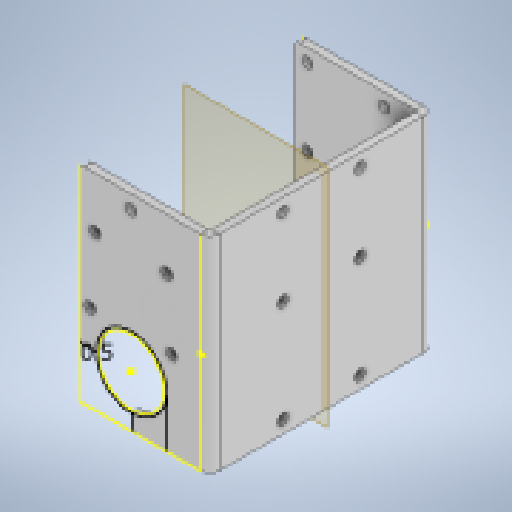
# Autodesk Inventor part: axis_3_top_frame
Saved by Autodesk Inventor 2024.1 (Build 281209000, 209)
## iProperties
Created: 2023-09-27
Part Number: axis_3_top_frame
Material: Aluminum 6061-AHC
Document SubType Name: Sheet Metal
Designer: chanh
Density: 2.7 g/cm^3
Sheet Metal Rule: Default_mm
Appearance: Aluminum - Dark
Author: chanh
Autodesk Inventor part; units mm, degrees
ref_plane "YZ Plane" through (0, 0, 0) normal (1, 0, 0) x (0, 1, 0)
ref_plane "XZ Plane" through (0, 0, 0) normal (0, 1, 0) x (-1, 0, 0)
ref_plane "XY Plane" through (0, 0, 0) normal (0, 0, 1) x (1, 0, 0)
sketch "Sketch1" plane through (0, 0, 0) normal (1, 0, 0) x (0, 1, 0)
  line L0 (20.05, 20.25) -> (-20.05, 20.25)
  line L1 (-20.05, 20.25) -> (-20.05, -20.25)
  line L2 (-20.05, -20.25) -> (20.05, -20.25)
  line L3 (20.05, -20.25) -> (20.05, 20.25)
  line L4 (20.05, 20.25) -> (-20.05, -20.25) construction
  line L5 (-20.05, 20.25) -> (20.05, -20.25) construction
  point P0 (0, 0)
  dimension "d0" = 40.1
  dimension "d1" = 40.5
  measures "d0" distance of L2.end L1.end
  measures "d1" distance of L1.end L0.end
extrude "Plate1" add sketch "Sketch1" along normal blind 1.5
sketch "Sketch2" plane through (0, 20.05, 20.25) normal (0, 0, 1) x (1, 0, 0)
  line L0 (0, -40.1) -> (0, 0)
  line L1 (0, 0) -> (-24, 0)
  line L2 (-24, 0) -> (-24, -40.1)
  line L3 (-24, -40.1) -> (0, -40.1)
  constraints: 6 end point, 1 horizontal, 1 perpendicular, 1 vertical
edge flange "Flange1" height 25.5 angle 90 thickness 1.5 bend radius 0.31 thickness toward (0, 0, 1) relief straight relief width 1.5 relief depth 0.75 corner gap 0.31 corner form 0 edges at (0, 0, 20.25) (0, 0, -20.25) wall of the first edge with corners at (0, -20.05, 20.25) (0, 20.05, 20.25) (-24, 20.05, 20.25) (-24, -20.05, 20.25)
bend "Bend1"
corner "Corner1"
sketch "Sketch3" plane through (-24, -20.05, 21.75) normal (0, 0, 1) x (1, 0, 0)
  circle A0 centre (10.07, 10) radius 6.4 projected
  line L0 (0, 0) -> (0, 40.1) projected
  line L1 (23.69, 0) -> (0, 0) projected
  line L2 (23.69, 0) -> (23.69, 40.1) projected
  circle A1 centre (10.07, 10) radius 6.9
  line L3 (3.17, 10) -> (0, 10)
  line L4 (16.97, 10) -> (16.97, 0)
  line L5 (10.07, 3.1) -> (10.07, 0)
  point P0 (24, 20.05)
  dimension "d13" = 0.5
  constraints: 6 end point, 3 point on circle, 3 point on line, 2 perpendicular, 1 centre point, 1 horizontal, 1 horizontal alignment, 1 tangent, 1 vertical alignment
  measures "d13" radial gap between concentric circles of A0 A1
sketch "Sketch4" plane through (-24, -20.05, -21.75) normal (0, 0, -1) x (-1, 0, 0)
  line L0 (-3.17, 10) -> (0, 10) projected
  line L1 (0, 0) -> (0, 40.1) projected
  circle A0 centre (-10.07, 10) radius 6.9 projected
  line L2 (-16.97, 10) -> (-16.97, 0) projected
  line L3 (-23.69, 0) -> (0, 0) projected
  line L4 (-10.07, 3.1) -> (-10.07, 0)
  point P0 (-24, 20.05)
  constraints: 2 end point, 1 perpendicular, 1 point on circle, 1 point on line, 1 vertical alignment
extrude "Cut1" cut sketch "Sketch3" against normal blind 1.5 contours A0 | L0 L3 A1 L5 L1 | A1
extrude "Cut2" cut sketch "Sketch4" against normal blind 1.5 contours A0 | L0 L1 L3 L4 A0
ref_plane "Work Plane1" through (-24, 20.05, 0) normal (0, 0, 1) x (1, 0, 0)
sketch "Sketch5" plane through (-24, 20.05, 21.75) normal (0, 0, 1) x (1, 0, 0)
  circle A0 centre (18.07, -23.2) radius 0.7835 projected
  circle A1 centre (2.07, -23.2) radius 0.7835 projected
  circle A2 centre (3.07, -9.98) radius 0.7835 projected
  circle A3 centre (17.07, -9.98) radius 0.7835 projected
  circle A4 centre (10.07, -2.68) radius 0.7835 projected
  point P0 (24, -20.05)
hole "Hole1" at (-13.93, 17.37, 21.75) at (-20.93, 10.07, 21.75) at (-6.93, 10.07, 21.75) at (-21.93, -3.15, 21.75) at (-5.93, -3.15, 21.75) direction (0, 0, -1) diameter 2.1 depth 1.5
sketch "Sketch6" plane through (-0.31, 20.05, -21.75) normal (0, 0, -1) x (-1, 0, 0)
  circle A0 centre (6.095, -17.6) radius 0.7835 projected
  circle A1 centre (6.095, -2.5) radius 0.7835 projected
  circle A2 centre (21.145, -2.5) radius 0.7835 projected
  circle A3 centre (21.145, -17.6) radius 0.7835 projected
  circle A4 centre (6.095, -37.6) radius 0.7835 projected
  point P0 (-0.31, -20.05)
fillet "Corner Round1" radius 1 6 edges at (-13.93, -20.05, -21) (-24, -10.05, -21) (-13.93, -20.05, 21) (-24, -10.05, 21) (-24, 20.05, 21) (-24, 20.05, -21)
hole "Hole3" at (-6.405, 17.55, -21.75) at (-21.455, 17.55, -21.75) at (-6.405, 2.45, -21.75) at (-21.455, 2.45, -21.75) at (-6.405, -17.55, -21.75) direction (0, 0, 1) diameter 2.1 depth 1.5
sketch "Sketch9" plane through (1.5, 0, 0) normal (1, 0, 0) x (0, 0, -1)
  circle A0 centre (7.525, 17.55) radius 0.7835
  circle A1 centre (-7.525, 17.55) radius 0.7835
  circle A2 centre (-7.525, 2.45) radius 0.7835
  circle A3 centre (7.525, 2.45) radius 0.7835
  circle A4 centre (7.525, -17.55) radius 0.7835
  circle A5 centre (-7.525, -17.55) radius 0.7835
  point P0 (0, 0)
  constraints: 6 centre point, 12 other
hole "Hole4" at (1.5, 17.55, 7.525) at (1.5, 17.55, -7.525) at (1.5, 2.45, 7.525) at (1.5, 2.45, -7.525) at (1.5, -17.55, 7.525) at (1.5, -17.55, -7.525) direction (-1, 0, 0) diameter 2.1 end through all
equation "\"d14\" = Thickness"
equation "\"d16\" = Thickness"
equation "\"d23\" = Thickness"
equation "\"d41\" = Thickness"
equation "\"d48\" = Thickness"
equation "\"d2\" = Thickness"
equation "\"d3\" = BendReliefWidth"
equation "\"d4\" = BendReliefDepth"
equation "\"d5\" = MinimumRemnant"
equation "\"d6\" = TransitionRadius"
equation "\"d9\" = BendRadius"
equation "\"d10\" = CornerReliefSize"
equation "\"d11\" = GapSize"
equation "\"d12\" = JacobiRadiusSize"
equation "\"BendReliefWidth\" = Thickness"
equation "\"BendReliefDepth\" = 0.5 * Thickness"
equation "\"CornerReliefSize\" = 4 * Thickness"
equation "\"MinimumRemnant\" = 2 * Thickness"
equation "\"TransitionRadius\" = BendRadius"
equation "\"JacobiRadiusSize\" = BendRadius"
equation "\"GapSize\" = Thickness"
equation "\"Thickness\" = 1.5"
equation "\"BendRadius\" = 0.31"
body "Solid1"
